Autodesk Fusion 360 part; units mm, degrees
note: some values were not read from the file. Chosen so that the rebuilt part matches the saved one: a direction. Set by a fixed rule: which sketch regions a step uses.
(part 2 of 6)
  spline S11 degree 5 poles (24.2977, -44.2586) (24.3025, -44.2616) (24.312, -44.2677) (24.3261, -44.2771) (24.3444, -44.2904) (24.3667, -44.3078) (24.3886, -44.326) (24.4101, -44.3445) (24.4315, -44.3633) (24.4529, -44.3822) (24.4741, -44.4013) (24.4952, -44.4206) (24.5161, -44.4401) (24.5367, -44.46) (24.5572, -44.4802) (24.5774, -44.5007) (24.5975, -44.5214) (24.6174, -44.5424) (24.6372, -44.5635) (24.6568, -44.5848) (24.6763, -44.6063) (24.6957, -44.6279) (24.715, -44.6497) (24.7341, -44.6718) (24.753, -44.694) (24.7719, -44.7164) (24.7905, -44.739) (24.8091, -44.7617) (24.8275, -44.7846) (24.8458, -44.8077) (24.864, -44.8309) (24.8821, -44.8542) (24.9, -44.8777) (24.9178, -44.9014) (24.9355, -44.9252) (24.9531, -44.9492) (24.9706, -44.9733) (24.9879, -44.9975) (25.0051, -45.0219) (25.0223, -45.0464) (25.0393, -45.0711) (25.0561, -45.0959) (25.0729, -45.1208) (25.0896, -45.1459) (25.1061, -45.171) (25.1225, -45.1963) (25.1389, -45.2218) (25.1551, -45.2473) (25.1712, -45.273) (25.1872, -45.2988) (25.203, -45.3247) (25.2188, -45.3508) (25.2345, -45.3769) (25.25, -45.4032) (25.2655, -45.4296) (25.2808, -45.4561) (25.2961, -45.4827) (25.3112, -45.5094) (25.3262, -45.5363) (25.3411, -45.5632) (25.3559, -45.5903) (25.3706, -45.6175) (25.3852, -45.6447) (25.3997, -45.6721) (25.4141, -45.6996) (25.4284, -45.7272) (25.4426, -45.7549) (25.4566, -45.7827) (25.4706, -45.8106) (25.4845, -45.8386) (25.4982, -45.8667) (25.5092, -45.8892) (25.5173, -45.9062) (25.5227, -45.9175) (25.5254, -45.9232) knots 0 0 0 0 0 0 0.01428571 0.02857143 0.04285714 0.05714286 0.07142857 0.08571429 0.1 0.11428571 0.12857143 0.14285714 0.15714286 0.17142857 0.18571429 0.2 0.21428571 0.22857143 0.24285714 0.25714286 0.27142857 0.28571429 0.3 0.31428571 0.32857143 0.34285714 0.35714286 0.37142857 0.38571429 0.4 0.41428571 0.42857143 0.44285714 0.45714286 0.47142857 0.48571429 0.5 0.51428571 0.52857143 0.54285714 0.55714286 0.57142857 0.58571429 0.6 0.61428571 0.62857143 0.64285714 0.65714286 0.67142857 0.68571429 0.7 0.71428571 0.72857143 0.74285714 0.75714286 0.77142857 0.78571429 0.8 0.81428571 0.82857143 0.84285714 0.85714286 0.87142857 0.88571429 0.9 0.91428571 0.92857143 0.94285714 0.95714286 0.97142857 0.98571429 1 1 1 1 1 1
  line L11 (24.2977, -44.2586) -> (23.8833, -44.0024)
  arc A23 (23.8504, -43.8655) -> (23.8833, -44.0024) centre (23.9359, -43.9173) ccw
  arc A24 (23.8504, -43.8655) -> (24.3428, -42.9686) centre (13.5, -37.5997) ccw
  arc A25 (24.4759, -42.923) -> (24.3428, -42.9686) centre (24.4324, -43.013) ccw
  line L12 (24.4759, -42.923) -> (24.9145, -43.135)
  spline S12 degree 5 poles (24.9145, -43.135) (24.9196, -43.1374) (24.9299, -43.1422) (24.9454, -43.149) (24.9664, -43.1574) (24.9931, -43.1668) (25.0201, -43.1755) (25.0473, -43.1838) (25.0747, -43.1918) (25.1021, -43.1996) (25.1296, -43.2072) (25.1572, -43.2147) (25.1849, -43.2218) (25.2128, -43.2286) (25.2408, -43.235) (25.2689, -43.2411) (25.2972, -43.2469) (25.3255, -43.2524) (25.354, -43.2578) (25.3825, -43.2629) (25.4111, -43.2679) (25.4398, -43.2726) (25.4685, -43.2771) (25.4974, -43.2814) (25.5263, -43.2855) (25.5553, -43.2893) (25.5844, -43.293) (25.6135, -43.2964) (25.6427, -43.2997) (25.672, -43.3027) (25.7014, -43.3056) (25.7308, -43.3083) (25.7602, -43.3108) (25.7898, -43.3132) (25.8194, -43.3153) (25.849, -43.3173) (25.8787, -43.3191) (25.9085, -43.3207) (25.9383, -43.3221) (25.9682, -43.3234) (25.9981, -43.3245) (26.0281, -43.3254) (26.0581, -43.3262) (26.0882, -43.3268) (26.1183, -43.3273) (26.1485, -43.3275) (26.1787, -43.3276) (26.209, -43.3276) (26.2393, -43.3274) (26.2696, -43.327) (26.3, -43.3265) (26.3305, -43.3259) (26.3609, -43.325) (26.3915, -43.3241) (26.422, -43.3229) (26.4526, -43.3216) (26.4832, -43.3202) (26.5139, -43.3186) (26.5446, -43.3169) (26.5754, -43.315) (26.6061, -43.313) (26.637, -43.3108) (26.6678, -43.3085) (26.6987, -43.306) (26.7296, -43.3034) (26.7605, -43.3006) (26.7915, -43.2977) (26.8225, -43.2947) (26.8536, -43.2915) (26.8846, -43.2881) (26.9157, -43.2847) (26.9406, -43.2818) (26.9593, -43.2795) (26.9718, -43.278) (26.978, -43.2772) knots 0 0 0 0 0 0 0.01428571 0.02857143 0.04285714 0.05714286 0.07142857 0.08571429 0.1 0.11428571 0.12857143 0.14285714 0.15714286 0.17142857 0.18571429 0.2 0.21428571 0.22857143 0.24285714 0.25714286 0.27142857 0.28571429 0.3 0.31428571 0.32857143 0.34285714 0.35714286 0.37142857 0.38571429 0.4 0.41428571 0.42857143 0.44285714 0.45714286 0.47142857 0.48571429 0.5 0.51428571 0.52857143 0.54285714 0.55714286 0.57142857 0.58571429 0.6 0.61428571 0.62857143 0.64285714 0.65714286 0.67142857 0.68571429 0.7 0.71428571 0.72857143 0.74285714 0.75714286 0.77142857 0.78571429 0.8 0.81428571 0.82857143 0.84285714 0.85714286 0.87142857 0.88571429 0.9 0.91428571 0.92857143 0.94285714 0.95714286 0.97142857 0.98571429 1 1 1 1 1 1
  arc A26 (26.978, -43.2772) -> (27.2699, -42.5272) centre (13.5, -37.5997) ccw
  spline S13 degree 5 poles (25.6532, -41.2371) (25.6586, -41.2387) (25.6694, -41.2421) (25.6854, -41.2476) (25.7066, -41.2557) (25.7326, -41.2668) (25.7584, -41.2786) (25.784, -41.2909) (25.8096, -41.3035) (25.8351, -41.3163) (25.8605, -41.3292) (25.8859, -41.3424) (25.9111, -41.3559) (25.9362, -41.3697) (25.9612, -41.3839) (25.9861, -41.3985) (26.0108, -41.4133) (26.0355, -41.4284) (26.06, -41.4437) (26.0845, -41.4592) (26.1089, -41.4749) (26.1333, -41.4908) (26.1575, -41.5069) (26.1817, -41.5232) (26.2057, -41.5398) (26.2297, -41.5565) (26.2536, -41.5735) (26.2774, -41.5907) (26.3011, -41.608) (26.3248, -41.6255) (26.3484, -41.6433) (26.3719, -41.6611) (26.3953, -41.6792) (26.4186, -41.6975) (26.4419, -41.7159) (26.465, -41.7345) (26.4881, -41.7532) (26.5112, -41.7722) (26.5341, -41.7913) (26.557, -41.8105) (26.5798, -41.8299) (26.6025, -41.8495) (26.6252, -41.8692) (26.6477, -41.8891) (26.6702, -41.9092) (26.6927, -41.9294) (26.715, -41.9497) (26.7373, -41.9702) (26.7595, -41.9908) (26.7816, -42.0116) (26.8036, -42.0325) (26.8256, -42.0536) (26.8475, -42.0748) (26.8693, -42.0962) (26.8911, -42.1177) (26.9128, -42.1393) (26.9344, -42.1611) (26.9559, -42.183) (26.9774, -42.205) (26.9987, -42.2272) (27.0201, -42.2495) (27.0413, -42.2719) (27.0624, -42.2945) (27.0835, -42.3172) (27.1045, -42.34) (27.1255, -42.363) (27.1463, -42.386) (27.1671, -42.4092) (27.1878, -42.4326) (27.2085, -42.456) (27.229, -42.4796) (27.2454, -42.4986) (27.2577, -42.5128) (27.2659, -42.5224) (27.2699, -42.5272) knots 0 0 0 0 0 0 0.01428571 0.02857143 0.04285714 0.05714286 0.07142857 0.08571429 0.1 0.11428571 0.12857143 0.14285714 0.15714286 0.17142857 0.18571429 0.2 0.21428571 0.22857143 0.24285714 0.25714286 0.27142857 0.28571429 0.3 0.31428571 0.32857143 0.34285714 0.35714286 0.37142857 0.38571429 0.4 0.41428571 0.42857143 0.44285714 0.45714286 0.47142857 0.48571429 0.5 0.51428571 0.52857143 0.54285714 0.55714286 0.57142857 0.58571429 0.6 0.61428571 0.62857143 0.64285714 0.65714286 0.67142857 0.68571429 0.7 0.71428571 0.72857143 0.74285714 0.75714286 0.77142857 0.78571429 0.8 0.81428571 0.82857143 0.84285714 0.85714286 0.87142857 0.88571429 0.9 0.91428571 0.92857143 0.94285714 0.95714286 0.97142857 0.98571429 1 1 1 1 1 1
  line L13 (25.6532, -41.2371) -> (25.1866, -41.0968)
  arc A27 (25.1194, -40.9731) -> (25.1866, -41.0968) centre (25.2154, -41.001) ccw
  arc A28 (25.1194, -40.9731) -> (25.3629, -39.9794) centre (13.5, -37.5997) ccw
  arc A29 (25.4796, -39.9008) -> (25.3629, -39.9794) centre (25.4609, -39.999) ccw
  line L14 (25.4796, -39.9008) -> (25.9582, -39.9921)
  spline S14 degree 5 poles (25.9582, -39.9921) (25.9638, -39.9931) (25.9749, -39.9951) (25.9917, -39.9977) (26.0141, -40.0003) (26.0424, -40.0025) (26.0707, -40.0039) (26.0991, -40.0048) (26.1276, -40.0055) (26.1561, -40.0059) (26.1847, -40.0062) (26.2132, -40.0062) (26.2419, -40.006) (26.2705, -40.0053) (26.2992, -40.0042) (26.328, -40.0028) (26.3568, -40.0011) (26.3856, -39.9991) (26.4145, -39.9969) (26.4434, -39.9945) (26.4723, -39.9919) (26.5012, -39.989) (26.5301, -39.986) (26.5591, -39.9827) (26.5881, -39.9791) (26.6171, -39.9753) (26.6461, -39.9713) (26.6752, -39.9671) (26.7042, -39.9627) (26.7333, -39.958) (26.7624, -39.9532) (26.7915, -39.9482) (26.8206, -39.943) (26.8498, -39.9376) (26.8789, -39.9321) (26.908, -39.9263) (26.9372, -39.9203) (26.9664, -39.9142) (26.9956, -39.9079) (27.0247, -39.9014) (27.0539, -39.8947) (27.0831, -39.8878) (27.1123, -39.8808) (27.1415, -39.8736) (27.1708, -39.8662) (27.2, -39.8587) (27.2292, -39.851) (27.2584, -39.8431) (27.2876, -39.8351) (27.3169, -39.8269) (27.3461, -39.8185) (27.3753, -39.81) (27.4045, -39.8013) (27.4338, -39.7924) (27.463, -39.7834) (27.4922, -39.7743) (27.5214, -39.765) (27.5506, -39.7555) (27.5798, -39.7459) (27.6091, -39.7361) (27.6383, -39.7262) (27.6675, -39.7161) (27.6967, -39.7059) (27.7258, -39.6955) (27.755, -39.6849) (27.7842, -39.6743) (27.8134, -39.6634) (27.8425, -39.6525) (27.8717, -39.6414) (27.9008, -39.6301) (27.93, -39.6187) (27.9533, -39.6095) (27.9707, -39.6025) (27.9824, -39.5978) (27.9882, -39.5954) knots 0 0 0 0 0 0 0.01428571 0.02857143 0.04285714 0.05714286 0.07142857 0.08571429 0.1 0.11428571 0.12857143 0.14285714 0.15714286 0.17142857 0.18571429 0.2 0.21428571 0.22857143 0.24285714 0.25714286 0.27142857 0.28571429 0.3 0.31428571 0.32857143 0.34285714 0.35714286 0.37142857 0.38571429 0.4 0.41428571 0.42857143 0.44285714 0.45714286 0.47142857 0.48571429 0.5 0.51428571 0.52857143 0.54285714 0.55714286 0.57142857 0.58571429 0.6 0.61428571 0.62857143 0.64285714 0.65714286 0.67142857 0.68571429 0.7 0.71428571 0.72857143 0.74285714 0.75714286 0.77142857 0.78571429 0.8 0.81428571 0.82857143 0.84285714 0.85714286 0.87142857 0.88571429 0.9 0.91428571 0.92857143 0.94285714 0.95714286 0.97142857 0.98571429 1 1 1 1 1 1
  arc A30 (27.9882, -39.5954) -> (28.076, -38.7953) centre (13.5, -37.5997) ccw
  spline S15 degree 5 poles (26.1805, -37.9677) (26.1862, -37.9679) (26.1975, -37.9683) (26.2144, -37.9695) (26.2369, -37.9718) (26.2649, -37.9758) (26.2929, -37.9805) (26.3208, -37.9858) (26.3488, -37.9913) (26.3767, -37.9971) (26.4046, -38.003) (26.4325, -38.0092) (26.4604, -38.0157) (26.4882, -38.0225) (26.516, -38.0298) (26.5438, -38.0374) (26.5716, -38.0453) (26.5993, -38.0535) (26.627, -38.0619) (26.6546, -38.0706) (26.6823, -38.0794) (26.7099, -38.0884) (26.7375, -38.0977) (26.765, -38.1073) (26.7925, -38.117) (26.82, -38.127) (26.8475, -38.1372) (26.875, -38.1476) (26.9024, -38.1583) (26.9297, -38.1691) (26.9571, -38.1801) (26.9844, -38.1913) (27.0117, -38.2027) (27.039, -38.2143) (27.0662, -38.226) (27.0934, -38.238) (27.1206, -38.2501) (27.1477, -38.2625) (27.1749, -38.275) (27.2019, -38.2876) (27.229, -38.3005) (27.256, -38.3135) (27.283, -38.3267) (27.3099, -38.3401) (27.3368, -38.3536) (27.3637, -38.3673) (27.3906, -38.3812) (27.4174, -38.3952) (27.4442, -38.4094) (27.4709, -38.4237) (27.4976, -38.4383) (27.5243, -38.4529) (27.551, -38.4677) (27.5776, -38.4827) (27.6041, -38.4978) (27.6307, -38.5131) (27.6572, -38.5286) (27.6836, -38.5441) (27.7101, -38.5599) (27.7365, -38.5758) (27.7628, -38.5918) (27.7891, -38.608) (27.8154, -38.6243) (27.8417, -38.6408) (27.8679, -38.6574) (27.894, -38.6741) (27.9201, -38.691) (27.9462, -38.708) (27.9723, -38.7252) (27.9983, -38.7425) (28.0242, -38.76) (28.045, -38.7741) (28.0605, -38.7847) (28.0709, -38.7918) (28.076, -38.7953) knots 0 0 0 0 0 0 0.01428571 0.02857143 0.04285714 0.05714286 0.07142857 0.08571429 0.1 0.11428571 0.12857143 0.14285714 0.15714286 0.17142857 0.18571429 0.2 0.21428571 0.22857143 0.24285714 0.25714286 0.27142857 0.28571429 0.3 0.31428571 0.32857143 0.34285714 0.35714286 0.37142857 0.38571429 0.4 0.41428571 0.42857143 0.44285714 0.45714286 0.47142857 0.48571429 0.5 0.51428571 0.52857143 0.54285714 0.55714286 0.57142857 0.58571429 0.6 0.61428571 0.62857143 0.64285714 0.65714286 0.67142857 0.68571429 0.7 0.71428571 0.72857143 0.74285714 0.75714286 0.77142857 0.78571429 0.8 0.81428571 0.82857143 0.84285714 0.85714286 0.87142857 0.88571429 0.9 0.91428571 0.92857143 0.94285714 0.95714286 0.97142857 0.98571429 1 1 1 1 1 1
  line L15 (26.1805, -37.9677) -> (25.6935, -37.9529)
  arc A31 (25.5966, -37.8509) -> (25.6935, -37.9529) centre (25.6966, -37.853) ccw
  arc A32 (25.5966, -37.8509) -> (25.5746, -36.828) centre (13.5, -37.5997) ccw
  arc A33 (25.667, -36.7218) -> (25.5746, -36.828) centre (25.6744, -36.8216) ccw
  line L16 (25.667, -36.7218) -> (26.1529, -36.6861)
  spline S16 degree 5 poles (26.1529, -36.6861) (26.1586, -36.6857) (26.1698, -36.6847) (26.1867, -36.6829) (26.209, -36.6796) (26.2369, -36.6744) (26.2646, -36.6684) (26.2923, -36.662) (26.32, -36.6552) (26.3476, -36.6483) (26.3753, -36.6412) (26.4029, -36.6338) (26.4305, -36.6261) (26.458, -36.6181) (26.4855, -36.6096) (26.5129, -36.6008) (26.5402, -36.5917) (26.5676, -36.5823) (26.5949, -36.5727) (26.6221, -36.5629) (26.6494, -36.5529) (26.6766, -36.5427) (26.7037, -36.5322) (26.7309, -36.5215) (26.7579, -36.5106) (26.785, -36.4994) (26.812, -36.488) (26.839, -36.4764) (26.8659, -36.4646) (26.8928, -36.4527) (26.9196, -36.4405) (26.9465, -36.4281) (26.9732, -36.4156) (27, -36.4028) (27.0267, -36.3899) (27.0533, -36.3768) (27.08, -36.3634) (27.1066, -36.35) (27.1331, -36.3363) (27.1596, -36.3225) (27.1861, -36.3085) (27.2125, -36.2943) (27.2389, -36.2799) (27.2652, -36.2654) (27.2916, -36.2508) (27.3178, -36.2359) (27.344, -36.2209) (27.3702, -36.2057) (27.3964, -36.1904) (27.4225, -36.1749) (27.4486, -36.1593) (27.4746, -36.1435) (27.5006, -36.1275) (27.5265, -36.1114) (27.5524, -36.0952) (27.5782, -36.0787) (27.6041, -36.0622) (27.6298, -36.0455) (27.6556, -36.0286) (27.6812, -36.0116) (27.7069, -35.9945) (27.7325, -35.9772) (27.758, -35.9597) (27.7835, -35.9421) (27.809, -35.9244) (27.8344, -35.9066) (27.8598, -35.8886) (27.8851, -35.8704) (27.9104, -35.8521) (27.9356, -35.8337) (27.9608, -35.8152) (27.9809, -35.8002) (27.996, -35.7889) (28.006, -35.7814) (28.011, -35.7776) knots 0 0 0 0 0 0 0.01428571 0.02857143 0.04285714 0.05714286 0.07142857 0.08571429 0.1 0.11428571 0.12857143 0.14285714 0.15714286 0.17142857 0.18571429 0.2 0.21428571 0.22857143 0.24285714 0.25714286 0.27142857 0.28571429 0.3 0.31428571 0.32857143 0.34285714 0.35714286 0.37142857 0.38571429 0.4 0.41428571 0.42857143 0.44285714 0.45714286 0.47142857 0.48571429 0.5 0.51428571 0.52857143 0.54285714 0.55714286 0.57142857 0.58571429 0.6 0.61428571 0.62857143 0.64285714 0.65714286 0.67142857 0.68571429 0.7 0.71428571 0.72857143 0.74285714 0.75714286 0.77142857 0.78571429 0.8 0.81428571 0.82857143 0.84285714 0.85714286 0.87142857 0.88571429 0.9 0.91428571 0.92857143 0.94285714 0.95714286 0.97142857 0.98571429 1 1 1 1 1 1
  arc A34 (28.011, -35.7776) -> (27.8888, -34.982) centre (13.5, -37.5997) ccw
  spline S17 degree 5 poles (25.8437, -34.6732) (25.8492, -34.6719) (25.8602, -34.6694) (25.8769, -34.6662) (25.8992, -34.6626) (25.9273, -34.6591) (25.9555, -34.6565) (25.9839, -34.6544) (26.0123, -34.6525) (26.0408, -34.6508) (26.0693, -34.6493) (26.0978, -34.648) (26.1264, -34.6471) (26.1551, -34.6465) (26.1838, -34.6463) (26.2126, -34.6465) (26.2415, -34.647) (26.2704, -34.6477) (26.2993, -34.6487) (26.3282, -34.6498) (26.3572, -34.6512) (26.3862, -34.6528) (26.4153, -34.6546) (26.4444, -34.6567) (26.4735, -34.659) (26.5026, -34.6616) (26.5318, -34.6643) (26.561, -34.6673) (26.5903, -34.6704) (26.6195, -34.6738) (26.6488, -34.6773) (26.6781, -34.6811) (26.7074, -34.685) (26.7367, -34.6892) (26.7661, -34.6935) (26.7954, -34.698) (26.8248, -34.7027) (26.8542, -34.7076) (26.8837, -34.7126) (26.9131, -34.7179) (26.9426, -34.7233) (26.972, -34.7289) (27.0015, -34.7347) (27.031, -34.7406) (27.0605, -34.7467) (27.09, -34.753) (27.1195, -34.7594) (27.1491, -34.766) (27.1786, -34.7728) (27.2082, -34.7797) (27.2377, -34.7868) (27.2673, -34.7941) (27.2968, -34.8015) (27.3264, -34.8091) (27.356, -34.8168) (27.3856, -34.8247) (27.4152, -34.8328) (27.4448, -34.841) (27.4744, -34.8493) (27.504, -34.8578) (27.5336, -34.8665) (27.5632, -34.8753) (27.5928, -34.8843) (27.6224, -34.8934) (27.652, -34.9027) (27.6816, -34.9121) (27.7112, -34.9216) (27.7408, -34.9313) (27.7704, -34.9412) (27.8, -34.9512) (27.8296, -34.9613) (27.8533, -34.9695) (27.8711, -34.9758) (27.8829, -34.9799) (27.8888, -34.982) knots 0 0 0 0 0 0 0.01428571 0.02857143 0.04285714 0.05714286 0.07142857 0.08571429 0.1 0.11428571 0.12857143 0.14285714 0.15714286 0.17142857 0.18571429 0.2 0.21428571 0.22857143 0.24285714 0.25714286 0.27142857 0.28571429 0.3 0.31428571 0.32857143 0.34285714 0.35714286 0.37142857 0.38571429 0.4 0.41428571 0.42857143 0.44285714 0.45714286 0.47142857 0.48571429 0.5 0.51428571 0.52857143 0.54285714 0.55714286 0.57142857 0.58571429 0.6 0.61428571 0.62857143 0.64285714 0.65714286 0.67142857 0.68571429 0.7 0.71428571 0.72857143 0.74285714 0.75714286 0.77142857 0.78571429 0.8 0.81428571 0.82857143 0.84285714 0.85714286 0.87142857 0.88571429 0.9 0.91428571 0.92857143 0.94285714 0.95714286 0.97142857 0.98571429 1 1 1 1 1 1
  line L17 (25.8437, -34.6732) -> (25.3695, -34.785)
  arc A35 (25.2494, -34.7115) -> (25.3695, -34.785) centre (25.3465, -34.6876) ccw
  arc A36 (25.2494, -34.7115) -> (24.9634, -33.7291) centre (13.5, -37.5997) ccw
  arc A37 (25.0252, -33.6027) -> (24.9634, -33.7291) centre (25.0581, -33.6971) ccw
  line L18 (25.0252, -33.6027) -> (25.4853, -33.4424)
  spline S18 degree 5 poles (25.4853, -33.4424) (25.4907, -33.4406) (25.5013, -33.4367) (25.5171, -33.4305) (25.5378, -33.4216) (25.5634, -33.4094) (25.5887, -33.3964) (25.6137, -33.383) (25.6387, -33.3694) (25.6636, -33.3555) (25.6885, -33.3415) (25.7133, -33.3272) (25.7379, -33.3127) (25.7624, -33.2977) (25.7867, -33.2825) (25.8109, -33.2669) (25.835, -33.251) (25.859, -33.2349) (25.8829, -33.2185) (25.9067, -33.202) (25.9304, -33.1853) (25.954, -33.1683) (25.9775, -33.1512) (26.001, -33.1339) (26.0243, -33.1163) (26.0475, -33.0985) (26.0707, -33.0805) (26.0937, -33.0623) (26.1167, -33.044) (26.1396, -33.0254) (26.1623, -33.0067) (26.185, -32.9878) (26.2077, -32.9688) (26.2302, -32.9495) (26.2526, -32.9301) (26.275, -32.9106) (26.2973, -32.8908) (26.3195, -32.8709) (26.3416, -32.8508) (26.3636, -32.8306) (26.3855, -32.8102) (26.4074, -32.7897) (26.4292, -32.769) (26.4509, -32.7482) (26.4725, -32.7272) (26.494, -32.7061) (26.5155, -32.6848) (26.5368, -32.6633) (26.5581, -32.6418) (26.5793, -32.6201) (26.6005, -32.5982) (26.6215, -32.5762) (26.6425, -32.5541) (26.6634, -32.5318) (26.6842, -32.5094) (26.7049, -32.4868) (26.7255, -32.4642) (26.7461, -32.4414) (26.7666, -32.4184) (26.787, -32.3953) (26.8073, -32.3721) (26.8276, -32.3488) (26.8477, -32.3254) (26.8678, -32.3018) (26.8878, -32.2781) (26.9078, -32.2542) (26.9276, -32.2303) (26.9474, -32.2062) (26.9671, -32.182) (26.9867, -32.1577) (27.0062, -32.1332) (27.0218, -32.1136) (27.0334, -32.0988) (27.0411, -32.0889) (27.045, -32.084) knots 0 0 0 0 0 0 0.01428571 0.02857143 0.04285714 0.05714286 0.07142857 0.08571429 0.1 0.11428571 0.12857143 0.14285714 0.15714286 0.17142857 0.18571429 0.2 0.21428571 0.22857143 0.24285714 0.25714286 0.27142857 0.28571429 0.3 0.31428571 0.32857143 0.34285714 0.35714286 0.37142857 0.38571429 0.4 0.41428571 0.42857143 0.44285714 0.45714286 0.47142857 0.48571429 0.5 0.51428571 0.52857143 0.54285714 0.55714286 0.57142857 0.58571429 0.6 0.61428571 0.62857143 0.64285714 0.65714286 0.67142857 0.68571429 0.7 0.71428571 0.72857143 0.74285714 0.75714286 0.77142857 0.78571429 0.8 0.81428571 0.82857143 0.84285714 0.85714286 0.87142857 0.88571429 0.9 0.91428571 0.92857143 0.94285714 0.95714286 0.97142857 0.98571429 1 1 1 1 1 1
  arc A38 (27.045, -32.084) -> (26.721, -31.3471) centre (13.5, -37.5997) ccw
  spline S19 degree 5 poles (24.6656, -31.5781) (24.6706, -31.5755) (24.6806, -31.5702) (24.6959, -31.5628) (24.7165, -31.5535) (24.7428, -31.5429) (24.7694, -31.5331) (24.7962, -31.5237) (24.8232, -31.5145) (24.8502, -31.5055) (24.8774, -31.4967) (24.9046, -31.4881) (24.932, -31.4797) (24.9596, -31.4718) (24.9873, -31.4642) (25.0151, -31.4569) (25.0431, -31.4499) (25.0712, -31.4431) (25.0994, -31.4365) (25.1277, -31.4302) (25.156, -31.424) (25.1844, -31.418) (25.213, -31.4123) (25.2416, -31.4067) (25.2703, -31.4014) (25.2991, -31.3963) (25.328, -31.3914) (25.357, -31.3868) (25.3861, -31.3822) (25.4152, -31.3779) (25.4444, -31.3738) (25.4736, -31.3698) (25.503, -31.366) (25.5324, -31.3624) (25.5619, -31.359) (25.5914, -31.3558) (25.621, -31.3527) (25.6507, -31.3498) (25.6804, -31.3471) (25.7102, -31.3445) (25.74, -31.3421) (25.7699, -31.3399) (25.7999, -31.3378) (25.8299, -31.3359) (25.86, -31.3342) (25.8901, -31.3326) (25.9203, -31.3312) (25.9506, -31.3299) (25.9809, -31.3288) (26.0112, -31.3279) (26.0416, -31.3271) (26.072, -31.3265) (26.1025, -31.326) (26.133, -31.3256) (26.1636, -31.3254) (26.1942, -31.3254) (26.2249, -31.3255) (26.2556, -31.3258) (26.2864, -31.3262) (26.3172, -31.3268) (26.348, -31.3275) (26.3789, -31.3283) (26.4098, -31.3293) (26.4408, -31.3305) (26.4717, -31.3317) (26.5028, -31.3332) (26.5339, -31.3347) (26.565, -31.3364) (26.5961, -31.3383) (26.6273, -31.3403) (26.6585, -31.3424) (26.6835, -31.3442) (26.7023, -31.3457) (26.7148, -31.3466) (26.721, -31.3471) knots 0 0 0 0 0 0 0.01428571 0.02857143 0.04285714 0.05714286 0.07142857 0.08571429 0.1 0.11428571 0.12857143 0.14285714 0.15714286 0.17142857 0.18571429 0.2 0.21428571 0.22857143 0.24285714 0.25714286 0.27142857 0.28571429 0.3 0.31428571 0.32857143 0.34285714 0.35714286 0.37142857 0.38571429 0.4 0.41428571 0.42857143 0.44285714 0.45714286 0.47142857 0.48571429 0.5 0.51428571 0.52857143 0.54285714 0.55714286 0.57142857 0.58571429 0.6 0.61428571 0.62857143 0.64285714 0.65714286 0.67142857 0.68571429 0.7 0.71428571 0.72857143 0.74285714 0.75714286 0.77142857 0.78571429 0.8 0.81428571 0.82857143 0.84285714 0.85714286 0.87142857 0.88571429 0.9 0.91428571 0.92857143 0.94285714 0.95714286 0.97142857 0.98571429 1 1 1 1 1 1
  line L19 (24.6656, -31.5781) -> (24.2365, -31.8088)
  arc A39 (24.1015, -31.7689) -> (24.2365, -31.8088) centre (24.1892, -31.7207) ccw
  arc A40 (24.1015, -31.7689) -> (23.571, -30.8941) centre (13.5, -37.5997) ccw
  arc A41 (23.598, -30.7559) -> (23.571, -30.8941) centre (23.6542, -30.8387) ccw
  line L20 (23.598, -30.7559) -> (24.0009, -30.4821)
  spline S20 degree 5 poles (24.0009, -30.4821) (24.0056, -30.4789) (24.0149, -30.4724) (24.0286, -30.4624) (24.0463, -30.4483) (24.0678, -30.4299) (24.0889, -30.4109) (24.1096, -30.3915) (24.1302, -30.3718) (24.1507, -30.3519) (24.1711, -30.332) (24.1913, -30.3118) (24.2113, -30.2913) (24.2311, -30.2706) (24.2507, -30.2495) (24.27, -30.2282) (24.2892, -30.2066) (24.3082, -30.1848) (24.327, -30.1629) (24.3457, -30.1408) (24.3643, -30.1185) (24.3827, -30.096) (24.401, -30.0734) (24.4192, -30.0505) (24.4371, -30.0275) (24.455, -30.0043) (24.4727, -29.981) (24.4902, -29.9574) (24.5077, -29.9338) (24.525, -29.9099) (24.5421, -29.886) (24.5592, -29.8619) (24.5761, -29.8376) (24.5929, -29.8132) (24.6095, -29.7886) (24.6261, -29.7639) (24.6425, -29.7391) (24.6587, -29.7141) (24.6749, -29.689) (24.6909, -29.6638) (24.7069, -29.6384) (24.7227, -29.6129) (24.7383, -29.5873) (24.7539, -29.5616) (24.7694, -29.5357) (24.7847, -29.5097) (24.7999, -29.4836) (24.815, -29.4574) (24.83, -29.431) (24.8448, -29.4046) (24.8596, -29.378) (24.8742, -29.3513) (24.8887, -29.3245) (24.9031, -29.2976) (24.9174, -29.2705) (24.9316, -29.2434) (24.9457, -29.2161) (24.9597, -29.1888) (24.9735, -29.1613) (24.9873, -29.1338) (25.0009, -29.1061) (25.0144, -29.0783) (25.0278, -29.0504) (25.0411, -29.0225) (25.0543, -28.9944) (25.0674, -28.9662) (25.0804, -28.9379) (25.0932, -28.9095) (25.106, -28.8811) (25.1186, -28.8525) (25.1312, -28.8238) (25.1411, -28.8008) (25.1485, -28.7835) (25.1534, -28.772) (25.1559, -28.7662) knots 0 0 0 0 0 0 0.01428571 0.02857143 0.04285714 0.05714286 0.07142857 0.08571429 0.1 0.11428571 0.12857143 0.14285714 0.15714286 0.17142857 0.18571429 0.2 0.21428571 0.22857143 0.24285714 0.25714286 0.27142857 0.28571429 0.3 0.31428571 0.32857143 0.34285714 0.35714286 0.37142857 0.38571429 0.4 0.41428571 0.42857143 0.44285714 0.45714286 0.47142857 0.48571429 0.5 0.51428571 0.52857143 0.54285714 0.55714286 0.57142857 0.58571429 0.6 0.61428571 0.62857143 0.64285714 0.65714286 0.67142857 0.68571429 0.7 0.71428571 0.72857143 0.74285714 0.75714286 0.77142857 0.78571429 0.8 0.81428571 0.82857143 0.84285714 0.85714286 0.87142857 0.88571429 0.9 0.91428571 0.92857143 0.94285714 0.95714286 0.97142857 0.98571429 1 1 1 1 1 1
  arc A42 (25.1559, -28.7662) -> (24.6523, -28.1383) centre (13.5, -37.5997) ccw
  spline S21 degree 5 poles (22.7267, -28.8934) (22.7308, -28.8896) (22.7391, -28.8819) (22.7519, -28.8708) (22.7694, -28.8565) (22.7921, -28.8395) (22.8152, -28.8231) (22.8387, -28.807) (22.8624, -28.7912) (22.8862, -28.7755) (22.9101, -28.7599) (22.9342, -28.7446) (22.9585, -28.7295) (22.9831, -28.7146) (23.0078, -28.7001) (23.0329, -28.6858) (23.0581, -28.6718) (23.0835, -28.658) (23.109, -28.6444) (23.1347, -28.6309) (23.1604, -28.6176) (23.1864, -28.6045) (23.2124, -28.5916) (23.2387, -28.5788) (23.265, -28.5663) (23.2915, -28.5539) (23.3182, -28.5417) (23.345, -28.5296) (23.3719, -28.5178) (23.3989, -28.506) (23.426, -28.4945) (23.4532, -28.4831) (23.4806, -28.4718) (23.5081, -28.4607) (23.5356, -28.4498) (23.5633, -28.439) (23.5911, -28.4284) (23.619, -28.4179) (23.6471, -28.4076) (23.6752, -28.3974) (23.7034, -28.3874) (23.7317, -28.3775) (23.7601, -28.3678) (23.7886, -28.3581) (23.8172, -28.3487) (23.8459, -28.3394) (23.8747, -28.3302) (23.9036, -28.3211) (23.9326, -28.3122) (23.9616, -28.3035) (23.9908, -28.2948) (24.02, -28.2863) (24.0493, -28.278) (24.0787, -28.2697) (24.1082, -28.2617) (24.1378, -28.2537) (24.1674, -28.2459) (24.1972, -28.2382) (24.227, -28.2306) (24.2569, -28.2232) (24.2868, -28.2159) (24.3169, -28.2087) (24.347, -28.2017) (24.3772, -28.1948) (24.4075, -28.188) (24.4378, -28.1813) (24.4682, -28.1748) (24.4987, -28.1684) (24.5293, -28.1621) (24.5599, -28.156) (24.5906, -28.15) (24.6152, -28.1452) (24.6337, -28.1418) (24.6461, -28.1395) (24.6523, -28.1383) knots 0 0 0 0 0 0 0.01428571 0.02857143 0.04285714 0.05714286 0.07142857 0.08571429 0.1 0.11428571 0.12857143 0.14285714 0.15714286 0.17142857 0.18571429 0.2 0.21428571 0.22857143 0.24285714 0.25714286 0.27142857 0.28571429 0.3 0.31428571 0.32857143 0.34285714 0.35714286 0.37142857 0.38571429 0.4 0.41428571 0.42857143 0.44285714 0.45714286 0.47142857 0.48571429 0.5 0.51428571 0.52857143 0.54285714 0.55714286 0.57142857 0.58571429 0.6 0.61428571 0.62857143 0.64285714 0.65714286 0.67142857 0.68571429 0.7 0.71428571 0.72857143 0.74285714 0.75714286 0.77142857 0.78571429 0.8 0.81428571 0.82857143 0.84285714 0.85714286 0.87142857 0.88571429 0.9 0.91428571 0.92857143 0.94285714 0.95714286 0.97142857 0.98571429 1 1 1 1 1 1
  line L21 (22.7267, -28.8934) -> (22.3719, -29.2273)
  arc A43 (22.2312, -29.2237) -> (22.3719, -29.2273) centre (22.3033, -29.1545) ccw
  arc A44 (22.2312, -29.2237) -> (21.4923, -28.516) centre (13.5, -37.5997) ccw
  arc A45 (21.4826, -28.3756) -> (21.4923, -28.516) centre (21.5583, -28.4409) ccw
  line L22 (21.4826, -28.3756) -> (21.8009, -28.0067)
  spline S22 degree 5 poles (21.8009, -28.0067) (21.8046, -28.0025) (21.8119, -27.9938) (21.8225, -27.9806) (21.836, -27.9624) (21.852, -27.9391) (21.8674, -27.9153) (21.8825, -27.8911) (21.8973, -27.8668) (21.9119, -27.8423) (21.9264, -27.8177) (21.9407, -27.793) (21.9548, -27.7681) (21.9685, -27.7429) (21.982, -27.7175) (21.9952, -27.6919) (22.0081, -27.6661) (22.0208, -27.6401) (22.0333, -27.6141) (22.0456, -27.5878) (22.0578, -27.5615) (22.0698, -27.535) (22.0816, -27.5084) (22.0932, -27.4817) (22.1046, -27.4548) (22.1159, -27.4278) (22.1269, -27.4006) (22.1378, -27.3734) (22.1485, -27.346) (22.159, -27.3185) (22.1694, -27.2909) (22.1796, -27.2632) (22.1897, -27.2354) (22.1996, -27.2075) (22.2093, -27.1794) (22.2189, -27.1513) (22.2283, -27.1231) (22.2376, -27.0947) (22.2467, -27.0663) (22.2557, -27.0378) (22.2645, -27.0091) (22.2731, -26.9804) (22.2816, -26.9516) (22.29, -26.9227) (22.2982, -26.8938) (22.3063, -26.8647) (22.3142, -26.8355) (22.322, -26.8063) (22.3297, -26.777) (22.3372, -26.7475) (22.3446, -26.7181) (22.3518, -26.6885) (22.3589, -26.6588) (22.3658, -26.6291) (22.3727, -26.5993) (22.3793, -26.5694) (22.3859, -26.5394) (22.3923, -26.5094) (22.3985, -26.4793) (22.4047, -26.4491) (22.4107, -26.4189) (22.4166, -26.3885) (22.4223, -26.3581) (22.4279, -26.3277) (22.4334, -26.2971) (22.4387, -26.2665) (22.4439, -26.2358) (22.449, -26.2051) (22.454, -26.1743) (22.4588, -26.1434) (22.4635, -26.1125) (22.4671, -26.0877) (22.4698, -26.0691) (22.4716, -26.0566) (22.4724, -26.0504) knots 0 0 0 0 0 0 0.01428571 0.02857143 0.04285714 0.05714286 0.07142857 0.08571429 0.1 0.11428571 0.12857143 0.14285714 0.15714286 0.17142857 0.18571429 0.2 0.21428571 0.22857143 0.24285714 0.25714286 0.27142857 0.28571429 0.3 0.31428571 0.32857143 0.34285714 0.35714286 0.37142857 0.38571429 0.4 0.41428571 0.42857143 0.44285714 0.45714286 0.47142857 0.48571429 0.5 0.51428571 0.52857143 0.54285714 0.55714286 0.57142857 0.58571429 0.6 0.61428571 0.62857143 0.64285714 0.65714286 0.67142857 0.68571429 0.7 0.71428571 0.72857143 0.74285714 0.75714286 0.77142857 0.78571429 0.8 0.81428571 0.82857143 0.84285714 0.85714286 0.87142857 0.88571429 0.9 0.91428571 0.92857143 0.94285714 0.95714286 0.97142857 0.98571429 1 1 1 1 1 1
  arc A46 (22.4724, -26.0504) -> (21.8235, -25.5743) centre (13.5, -37.5997) ccw
  spline S23 degree 5 poles (20.1589, -26.8021) (20.1619, -26.7972) (20.168, -26.7877) (20.1774, -26.7736) (20.1907, -26.7553) (20.2081, -26.733) (20.2262, -26.7112) (20.2448, -26.6896) (20.2635, -26.6682) (20.2825, -26.6468) (20.3016, -26.6256) (20.3209, -26.6046) (20.3404, -26.5837) (20.3603, -26.563) (20.3805, -26.5425) (20.401, -26.5223) (20.4217, -26.5022) (20.4426, -26.4823) (20.4638, -26.4625) (20.4851, -26.4429) (20.5065, -26.4234) (20.5282, -26.404) (20.55, -26.3847) (20.572, -26.3656) (20.5943, -26.3467) (20.6167, -26.3279) (20.6392, -26.3092) (20.662, -26.2906) (20.6849, -26.2722) (20.7079, -26.2539) (20.7312, -26.2357) (20.7545, -26.2176) (20.778, -26.1997) (20.8017, -26.1819) (20.8255, -26.1642) (20.8495, -26.1466) (20.8736, -26.1291) (20.8978, -26.1118) (20.9222, -26.0946) (20.9467, -26.0775) (20.9714, -26.0605) (20.9962, -26.0436) (21.0211, -26.0268) (21.0461, -26.0102) (21.0713, -25.9936) (21.0966, -25.9772) (21.1221, -25.9609) (21.1476, -25.9446) (21.1733, -25.9285) (21.1991, -25.9126) (21.225, -25.8967) (21.2511, -25.8809) (21.2772, -25.8652) (21.3035, -25.8497) (21.3299, -25.8342) (21.3564, -25.8189) (21.383, -25.8037) (21.4097, -25.7885) (21.4366, -25.7735) (21.4635, -25.7586) (21.4906, -25.7438) (21.5177, -25.7291) (21.545, -25.7145) (21.5724, -25.7) (21.5999, -25.6856) (21.6275, -25.6713) (21.6552, -25.6572) (21.683, -25.6431) (21.7109, -25.6291) (21.7388, -25.6153) (21.7669, -25.6015) (21.7895, -25.5906) (21.8065, -25.5824) (21.8178, -25.577) (21.8235, -25.5743) knots 0 0 0 0 0 0 0.01428571 0.02857143 0.04285714 0.05714286 0.07142857 0.08571429 0.1 0.11428571 0.12857143 0.14285714 0.15714286 0.17142857 0.18571429 0.2 0.21428571 0.22857143 0.24285714 0.25714286 0.27142857 0.28571429 0.3 0.31428571 0.32857143 0.34285714 0.35714286 0.37142857 0.38571429 0.4 0.41428571 0.42857143 0.44285714 0.45714286 0.47142857 0.48571429 0.5 0.51428571 0.52857143 0.54285714 0.55714286 0.57142857 0.58571429 0.6 0.61428571 0.62857143 0.64285714 0.65714286 0.67142857 0.68571429 0.7 0.71428571 0.72857143 0.74285714 0.75714286 0.77142857 0.78571429 0.8 0.81428571 0.82857143 0.84285714 0.85714286 0.87142857 0.88571429 0.9 0.91428571 0.92857143 0.94285714 0.95714286 0.97142857 0.98571429 1 1 1 1 1 1
  line L23 (20.1589, -26.8021) -> (19.9026, -27.2164)
  arc A47 (19.7658, -27.2493) -> (19.9026, -27.2164) centre (19.8176, -27.1638) ccw
  arc A48 (19.7658, -27.2493) -> (18.8689, -26.757) centre (13.5, -37.5997) ccw
  arc A49 (18.8233, -26.6238) -> (18.8689, -26.757) centre (18.9133, -26.6673) ccw
  line L24 (18.8233, -26.6238) -> (19.0352, -26.1852)
  spline S24 degree 5 poles (19.0352, -26.1852) (19.0377, -26.1801) (19.0425, -26.1698) (19.0493, -26.1543) (19.0577, -26.1333) (19.0671, -26.1066) (19.0758, -26.0796) (19.0841, -26.0524) (19.0921, -26.025) (19.0999, -25.9976) (19.1075, -25.9701) (19.115, -25.9425) (19.1221, -25.9148) (19.1289, -25.8869) (19.1353, -25.8589) (19.1414, -25.8308) (19.1472, -25.8025) (19.1527, -25.7742) (19.158, -25.7457) (19.1632, -25.7172) (19.1681, -25.6886) (19.1729, -25.6599) (19.1774, -25.6312) (19.1817, -25.6023) (19.1857, -25.5734) (19.1896, -25.5444) (19.1932, -25.5153) (19.1967, -25.4862) (19.1999, -25.457) (19.203, -25.4277) (19.2059, -25.3984) (19.2086, -25.3689) (19.2111, -25.3395) (19.2134, -25.3099) (19.2156, -25.2804) (19.2176, -25.2507) (19.2193, -25.221) (19.221, -25.1912) (19.2224, -25.1614) (19.2237, -25.1315) (19.2248, -25.1016) (19.2257, -25.0716) (19.2265, -25.0416) (19.2271, -25.0115) (19.2275, -24.9814) (19.2278, -24.9512) (19.2279, -24.921) (19.2279, -24.8907) (19.2277, -24.8604) (19.2273, -24.8301) (19.2268, -24.7997) (19.2261, -24.7693) (19.2253, -24.7388) (19.2243, -24.7083) (19.2232, -24.6777) (19.2219, -24.6471) (19.2205, -24.6165) (19.2189, -24.5858) (19.2172, -24.5551) (19.2153, -24.5244) (19.2132, -24.4936) (19.2111, -24.4628) (19.2087, -24.4319) (19.2063, -24.401) (19.2036, -24.3701) (19.2009, -24.3392) (19.198, -24.3082) (19.1949, -24.2772) (19.1917, -24.2462) (19.1884, -24.2151) (19.1849, -24.184) (19.182, -24.1591) (19.1798, -24.1404) (19.1783, -24.128) (19.1775, -24.1217) knots 0 0 0 0 0 0 0.01428571 0.02857143 0.04285714 0.05714286 0.07142857 0.08571429 0.1 0.11428571 0.12857143 0.14285714 0.15714286 0.17142857 0.18571429 0.2 0.21428571 0.22857143 0.24285714 0.25714286 0.27142857 0.28571429 0.3 0.31428571 0.32857143 0.34285714 0.35714286 0.37142857 0.38571429 0.4 0.41428571 0.42857143 0.44285714 0.45714286 0.47142857 0.48571429 0.5 0.51428571 0.52857143 0.54285714 0.55714286 0.57142857 0.58571429 0.6 0.61428571 0.62857143 0.64285714 0.65714286 0.67142857 0.68571429 0.7 0.71428571 0.72857143 0.74285714 0.75714286 0.77142857 0.78571429 0.8 0.81428571 0.82857143 0.84285714 0.85714286 0.87142857 0.88571429 0.9 0.91428571 0.92857143 0.94285714 0.95714286 0.97142857 0.98571429 1 1 1 1 1 1
  arc A50 (19.1775, -24.1217) -> (18.4274, -23.8298) centre (13.5, -37.5997) ccw
  spline S25 degree 5 poles (17.1374, -25.4465) (17.139, -25.4411) (17.1424, -25.4303) (17.1479, -25.4143) (17.1559, -25.3931) (17.167, -25.3671) (17.1789, -25.3413) (17.1912, -25.3157) (17.2038, -25.2901) (17.2166, -25.2646) (17.2295, -25.2392) (17.2427, -25.2138) (17.2562, -25.1886) (17.27, -25.1635) (17.2842, -25.1385) (17.2988, -25.1136) (17.3136, -25.0889) (17.3287, -25.0642) (17.344, -25.0397) (17.3595, -25.0152) (17.3751, -24.9908) (17.391, -24.9664) (17.4071, -24.9422) (17.4235, -24.9181) (17.44, -24.894) (17.4568, -24.87) (17.4738, -24.8461) (17.4909, -24.8223) (17.5083, -24.7986) (17.5258, -24.7749) (17.5435, -24.7514) (17.5614, -24.7279) (17.5795, -24.7044) (17.5977, -24.6811) (17.6162, -24.6579) (17.6348, -24.6347) (17.6535, -24.6116) (17.6725, -24.5885) (17.6916, -24.5656) (17.7108, -24.5427) (17.7302, -24.5199) (17.7498, -24.4972) (17.7695, -24.4745) (17.7894, -24.452) (17.8095, -24.4295) (17.8296, -24.4071) (17.85, -24.3847) (17.8705, -24.3624) (17.8911, -24.3402) (17.9119, -24.3181) (17.9328, -24.2961) (17.9539, -24.2741) (17.9751, -24.2522) (17.9965, -24.2304) (18.0179, -24.2086) (18.0396, -24.1869) (18.0613, -24.1653) (18.0832, -24.1438) (18.1053, -24.1224) (18.1275, -24.101) (18.1498, -24.0797) (18.1722, -24.0584) (18.1948, -24.0373) (18.2175, -24.0162) (18.2403, -23.9952) (18.2632, -23.9742) (18.2863, -23.9534) (18.3095, -23.9326) (18.3329, -23.9119) (18.3563, -23.8912) (18.3799, -23.8707) (18.3989, -23.8543) (18.4131, -23.842) (18.4227, -23.8339) (18.4274, -23.8298) knots 0 0 0 0 0 0 0.01428571 0.02857143 0.04285714 0.05714286 0.07142857 0.08571429 0.1 0.11428571 0.12857143 0.14285714 0.15714286 0.17142857 0.18571429 0.2 0.21428571 0.22857143 0.24285714 0.25714286 0.27142857 0.28571429 0.3 0.31428571 0.32857143 0.34285714 0.35714286 0.37142857 0.38571429 0.4 0.41428571 0.42857143 0.44285714 0.45714286 0.47142857 0.48571429 0.5 0.51428571 0.52857143 0.54285714 0.55714286 0.57142857 0.58571429 0.6 0.61428571 0.62857143 0.64285714 0.65714286 0.67142857 0.68571429 0.7 0.71428571 0.72857143 0.74285714 0.75714286 0.77142857 0.78571429 0.8 0.81428571 0.82857143 0.84285714 0.85714286 0.87142857 0.88571429 0.9 0.91428571 0.92857143 0.94285714 0.95714286 0.97142857 0.98571429 1 1 1 1 1 1
  line L25 (17.1374, -25.4465) -> (16.9971, -25.9131)
  arc A51 (16.8734, -25.9803) -> (16.9971, -25.9131) centre (16.9013, -25.8843) ccw
  arc A52 (16.8734, -25.9803) -> (15.8797, -25.7368) centre (13.5, -37.5997) ccw
  arc A53 (15.8011, -25.6201) -> (15.8797, -25.7368) centre (15.8993, -25.6388) ccw
  line L26 (15.8011, -25.6201) -> (15.8923, -25.1415)
  spline S26 degree 5 poles (15.8923, -25.1415) (15.8934, -25.1359) (15.8954, -25.1248) (15.8979, -25.108) (15.9006, -25.0856) (15.9028, -25.0573) (15.9042, -25.029) (15.9051, -25.0006) (15.9058, -24.9721) (15.9062, -24.9436) (15.9065, -24.9151) (15.9065, -24.8865) (15.9062, -24.8579) (15.9056, -24.8292) (15.9045, -24.8005) (15.9031, -24.7717) (15.9014, -24.7429) (15.8994, -24.7141) (15.8972, -24.6852) (15.8948, -24.6564) (15.8922, -24.6275) (15.8893, -24.5985) (15.8863, -24.5696) (15.8829, -24.5406) (15.8794, -24.5116) (15.8756, -24.4826) (15.8716, -24.4536) (15.8674, -24.4245) (15.8629, -24.3955) (15.8583, -24.3664) (15.8535, -24.3373) (15.8485, -24.3082) (15.8433, -24.2791) (15.8379, -24.25) (15.8323, -24.2208) (15.8266, -24.1917) (15.8206, -24.1625) (15.8145, -24.1333) (15.8081, -24.1042) (15.8016, -24.075) (15.795, -24.0458) (15.7881, -24.0166) (15.7811, -23.9874) (15.7739, -23.9582) (15.7665, -23.929) (15.759, -23.8997) (15.7513, -23.8705) (15.7434, -23.8413) (15.7354, -23.8121) (15.7272, -23.7829) (15.7188, -23.7536) (15.7103, -23.7244) (15.7016, -23.6952) (15.6927, -23.666) (15.6837, -23.6367) (15.6746, -23.6075) (15.6653, -23.5783) (15.6558, -23.5491) (15.6462, -23.5199) (15.6364, -23.4907) (15.6265, -23.4615) (15.6164, -23.4323) (15.6061, -23.4031) (15.5958, -23.3739) (15.5852, -23.3447) (15.5746, -23.3155) (15.5637, -23.2864) (15.5528, -23.2572) (15.5416, -23.228) (15.5304, -23.1989) (15.519, -23.1698) (15.5097, -23.1465) (15.5028, -23.129) (15.4981, -23.1173) (15.4957, -23.1115) knots 0 0 0 0 0 0 0.01428571 0.02857143 0.04285714 0.05714286 0.07142857 0.08571429 0.1 0.11428571 0.12857143 0.14285714 0.15714286 0.17142857 0.18571429 0.2 0.21428571 0.22857143 0.24285714 0.25714286 0.27142857 0.28571429 0.3 0.31428571 0.32857143 0.34285714 0.35714286 0.37142857 0.38571429 0.4 0.41428571 0.42857143 0.44285714 0.45714286 0.47142857 0.48571429 0.5 0.51428571 0.52857143 0.54285714 0.55714286 0.57142857 0.58571429 0.6 0.61428571 0.62857143 0.64285714 0.65714286 0.67142857 0.68571429 0.7 0.71428571 0.72857143 0.74285714 0.75714286 0.77142857 0.78571429 0.8 0.81428571 0.82857143 0.84285714 0.85714286 0.87142857 0.88571429 0.9 0.91428571 0.92857143 0.94285714 0.95714286 0.97142857 0.98571429 1 1 1 1 1 1
  arc A54 (15.4957, -23.1115) -> (14.6956, -23.0237) centre (13.5, -37.5997) ccw
  spline S27 degree 5 poles (13.868, -24.9192) (13.8681, -24.9135) (13.8686, -24.9022) (13.8698, -24.8853) (13.8721, -24.8628) (13.876, -24.8348) (13.8808, -24.8068) (13.8861, -24.7789) (13.8916, -24.7509) (13.8974, -24.723) (13.9033, -24.6951) (13.9095, -24.6672) (13.9159, -24.6393) (13.9228, -24.6115) (13.9301, -24.5837) (13.9377, -24.5559) (13.9456, -24.5282) (13.9538, -24.5005) (13.9622, -24.4728) (13.9708, -24.4451) (13.9797, -24.4175) (13.9887, -24.3898) (13.998, -24.3623) (14.0075, -24.3347) (14.0173, -24.3072) (14.0273, -24.2797) (14.0375, -24.2522) (14.0479, -24.2248) (14.0585, -24.1974) (14.0694, -24.17) (14.0804, -24.1426) (14.0916, -24.1153) (14.103, -24.088) (14.1145, -24.0607) (14.1263, -24.0335) (14.1383, -24.0063) (14.1504, -23.9791) (14.1627, -23.952) (14.1753, -23.9249) (14.1879, -23.8978) (14.2008, -23.8707) (14.2138, -23.8437) (14.227, -23.8167) (14.2404, -23.7898) (14.2539, -23.7629) (14.2676, -23.736) (14.2815, -23.7091) (14.2955, -23.6823) (14.3097, -23.6555) (14.324, -23.6288) (14.3385, -23.6021) (14.3532, -23.5754) (14.368, -23.5488) (14.383, -23.5221) (14.3981, -23.4956) (14.4134, -23.469) (14.4288, -23.4425) (14.4444, -23.4161) (14.4602, -23.3896) (14.476, -23.3633) (14.4921, -23.3369) (14.5083, -23.3106) (14.5246, -23.2843) (14.541, -23.2581) (14.5576, -23.2319) (14.5744, -23.2057) (14.5913, -23.1796) (14.6083, -23.1535) (14.6255, -23.1274) (14.6428, -23.1014) (14.6603, -23.0755) (14.6743, -23.0547) (14.685, -23.0392) (14.6921, -23.0288) (14.6956, -23.0237) knots 0 0 0 0 0 0 0.01428571 0.02857143 0.04285714 0.05714286 0.07142857 0.08571429 0.1 0.11428571 0.12857143 0.14285714 0.15714286 0.17142857 0.18571429 0.2 0.21428571 0.22857143 0.24285714 0.25714286 0.27142857 0.28571429 0.3 0.31428571 0.32857143 0.34285714 0.35714286 0.37142857 0.38571429 0.4 0.41428571 0.42857143 0.44285714 0.45714286 0.47142857 0.48571429 0.5 0.51428571 0.52857143 0.54285714 0.55714286 0.57142857 0.58571429 0.6 0.61428571 0.62857143 0.64285714 0.65714286 0.67142857 0.68571429 0.7 0.71428571 0.72857143 0.74285714 0.75714286 0.77142857 0.78571429 0.8 0.81428571 0.82857143 0.84285714 0.85714286 0.87142857 0.88571429 0.9 0.91428571 0.92857143 0.94285714 0.95714286 0.97142857 0.98571429 1 1 1 1 1 1
  line L27 (13.868, -24.9192) -> (13.8532, -25.4062)
  arc A55 (13.7512, -25.5031) -> (13.8532, -25.4062) centre (13.7532, -25.4031) ccw
  arc A56 (13.7512, -25.5031) -> (12.7282, -25.5252) centre (13.5, -37.5997) ccw
  arc A57 (12.6221, -25.4327) -> (12.7282, -25.5252) centre (12.7219, -25.4254) ccw
  line L28 (12.6221, -25.4327) -> (12.5864, -24.9468)
  spline S28 degree 5 poles (12.5864, -24.9468) (12.586, -24.9412) (12.585, -24.9299) (12.5831, -24.913) (12.5799, -24.8907) (12.5747, -24.8628) (12.5687, -24.8351) (12.5623, -24.8074) (12.5555, -24.7797) (12.5486, -24.7521) (12.5415, -24.7244) (12.5341, -24.6968) (12.5264, -24.6692) (12.5183, -24.6417) (12.5099, -24.6143) (12.5011, -24.5868) (12.492, -24.5595) (12.4826, -24.5321) (12.473, -24.5048) (12.4632, -24.4776) (12.4532, -24.4503) (12.443, -24.4231) (12.4325, -24.396) (12.4218, -24.3689) (12.4109, -24.3418) (12.3997, -24.3147) (12.3883, -24.2877) (12.3767, -24.2608) (12.3649, -24.2338) (12.3529, -24.2069) (12.3408, -24.1801) (12.3284, -24.1533) (12.3158, -24.1265) (12.3031, -24.0997) (12.2902, -24.073) (12.277, -24.0464) (12.2637, -24.0198) (12.2502, -23.9932) (12.2366, -23.9666) (12.2228, -23.9401) (12.2088, -23.9136) (12.1946, -23.8872) (12.1802, -23.8608) (12.1657, -23.8345) (12.151, -23.8082) (12.1362, -23.7819) (12.1212, -23.7557) (12.106, -23.7295) (12.0907, -23.7033) (12.0752, -23.6772) (12.0596, -23.6512) (12.0438, -23.6251) (12.0278, -23.5992) (12.0117, -23.5732) (11.9954, -23.5473) (11.979, -23.5215) (11.9625, -23.4957) (11.9458, -23.4699) (11.9289, -23.4442) (11.9119, -23.4185) (11.8947, -23.3928) (11.8774, -23.3672) (11.86, -23.3417) (11.8424, -23.3162) (11.8247, -23.2907) (11.8068, -23.2653) (11.7888, -23.2399) (11.7707, -23.2146) (11.7524, -23.1893) (11.734, -23.1641) (11.7154, -23.1389) (11.7005, -23.1188) (11.6892, -23.1037) (11.6817, -23.0937) (11.6779, -23.0887) knots 0 0 0 0 0 0 0.01428571 0.02857143 0.04285714 0.05714286 0.07142857 0.08571429 0.1 0.11428571 0.12857143 0.14285714 0.15714286 0.17142857 0.18571429 0.2 0.21428571 0.22857143 0.24285714 0.25714286 0.27142857 0.28571429 0.3 0.31428571 0.32857143 0.34285714 0.35714286 0.37142857 0.38571429 0.4 0.41428571 0.42857143 0.44285714 0.45714286 0.47142857 0.48571429 0.5 0.51428571 0.52857143 0.54285714 0.55714286 0.57142857 0.58571429 0.6 0.61428571 0.62857143 0.64285714 0.65714286 0.67142857 0.68571429 0.7 0.71428571 0.72857143 0.74285714 0.75714286 0.77142857 0.78571429 0.8 0.81428571 0.82857143 0.84285714 0.85714286 0.87142857 0.88571429 0.9 0.91428571 0.92857143 0.94285714 0.95714286 0.97142857 0.98571429 1 1 1 1 1 1
  arc A58 (11.6779, -23.0887) -> (10.8823, -23.2109) centre (13.5, -37.5997) ccw
  spline S29 degree 5 poles (10.5735, -25.256) (10.5722, -25.2505) (10.5697, -25.2395) (10.5664, -25.2229) (10.5629, -25.2005) (10.5594, -25.1724) (10.5568, -25.1442) (10.5546, -25.1158) (10.5528, -25.0874) (10.5511, -25.0589) (10.5496, -25.0304) (10.5483, -25.0019) (10.5474, -24.9733) (10.5468, -24.9446) (10.5466, -24.9159) (10.5468, -24.8871) (10.5473, -24.8582) (10.548, -24.8293) (10.549, -24.8004) (10.5501, -24.7715) (10.5515, -24.7425) (10.5531, -24.7135) (10.5549, -24.6844) (10.557, -24.6553) (10.5593, -24.6262) (10.5618, -24.5971) (10.5646, -24.5679) (10.5676, -24.5387) (10.5707, -24.5095) (10.5741, -24.4802) (10.5776, -24.4509) (10.5814, -24.4217) (10.5853, -24.3923) (10.5894, -24.363) (10.5938, -24.3336) (10.5983, -24.3043) (10.603, -24.2749) (10.6079, -24.2455) (10.6129, -24.2161) (10.6182, -24.1866) (10.6236, -24.1572) (10.6292, -24.1277) (10.6349, -24.0982) (10.6409, -24.0687) (10.647, -24.0392) (10.6533, -24.0097) (10.6597, -23.9802) (10.6663, -23.9507) (10.6731, -23.9211) (10.68, -23.8916) (10.6871, -23.862) (10.6944, -23.8324) (10.7018, -23.8029) (10.7094, -23.7733) (10.7171, -23.7437) (10.725, -23.7141) (10.733, -23.6845) (10.7413, -23.6549) (10.7496, -23.6253) (10.7581, -23.5957) (10.7668, -23.5661) (10.7756, -23.5365) (10.7846, -23.5069) (10.7937, -23.4773) (10.8029, -23.4477) (10.8123, -23.4181) (10.8219, -23.3885) (10.8316, -23.3589) (10.8415, -23.3293) (10.8514, -23.2997) (10.8616, -23.2701) (10.8698, -23.2464) (10.876, -23.2286) (10.8802, -23.2168) (10.8823, -23.2109) knots 0 0 0 0 0 0 0.01428571 0.02857143 0.04285714 0.05714286 0.07142857 0.08571429 0.1 0.11428571 0.12857143 0.14285714 0.15714286 0.17142857 0.18571429 0.2 0.21428571 0.22857143 0.24285714 0.25714286 0.27142857 0.28571429 0.3 0.31428571 0.32857143 0.34285714 0.35714286 0.37142857 0.38571429 0.4 0.41428571 0.42857143 0.44285714 0.45714286 0.47142857 0.48571429 0.5 0.51428571 0.52857143 0.54285714 0.55714286 0.57142857 0.58571429 0.6 0.61428571 0.62857143 0.64285714 0.65714286 0.67142857 0.68571429 0.7 0.71428571 0.72857143 0.74285714 0.75714286 0.77142857 0.78571429 0.8 0.81428571 0.82857143 0.84285714 0.85714286 0.87142857 0.88571429 0.9 0.91428571 0.92857143 0.94285714 0.95714286 0.97142857 0.98571429 1 1 1 1 1 1
  line L29 (10.5735, -25.256) -> (10.6852, -25.7303)
  arc A59 (10.6118, -25.8503) -> (10.6852, -25.7303) centre (10.5879, -25.7532) ccw
  arc A60 (10.6118, -25.8503) -> (9.6294, -26.1363) centre (13.5, -37.5997) ccw
  arc A61 (9.503, -26.0745) -> (9.6294, -26.1363) centre (9.5974, -26.0416) ccw
  line L30 (9.503, -26.0745) -> (9.3427, -25.6144)
  spline S30 degree 5 poles (9.3427, -25.6144) (9.3408, -25.6091) (9.337, -25.5984) (9.3308, -25.5826) (9.3219, -25.5619) (9.3097, -25.5363) (9.2967, -25.5111) (9.2833, -25.486) (9.2696, -25.461) (9.2558, -25.4361) (9.2418, -25.4112) (9.2275, -25.3865) (9.2129, -25.3618) (9.198, -25.3373) (9.1828, -25.313) (9.1672, -25.2888) (9.1513, -25.2647) (9.1351, -25.2407) (9.1188, -25.2168) (9.1023, -25.193) (9.0856, -25.1693) (9.0686, -25.1457) (9.0515, -25.1222) (9.0341, -25.0987) (9.0166, -25.0754) (8.9988, -25.0522) (8.9808, -25.029) (8.9626, -25.006) (8.9443, -24.983) (8.9257, -24.9602) (8.907, -24.9374) (8.8881, -24.9147) (8.8691, -24.8921) (8.8498, -24.8695) (8.8304, -24.8471) (8.8108, -24.8247) (8.7911, -24.8024) (8.7712, -24.7803) (8.7511, -24.7582) (8.7309, -24.7361) (8.7105, -24.7142) (8.69, -24.6923) (8.6693, -24.6705) (8.6485, -24.6489) (8.6275, -24.6272) (8.6063, -24.6057) (8.5851, -24.5843) (8.5636, -24.5629) (8.5421, -24.5416) (8.5203, -24.5204) (8.4985, -24.4993) (8.4765, -24.4782) (8.4544, -24.4573) (8.4321, -24.4364) (8.4097, -24.4156) (8.3871, -24.3948) (8.3645, -24.3742) (8.3416, -24.3536) (8.3187, -24.3331) (8.2956, -24.3127) (8.2724, -24.2924) (8.2491, -24.2722) (8.2256, -24.252) (8.2021, -24.2319) (8.1784, -24.2119) (8.1545, -24.192) (8.1306, -24.1721) (8.1065, -24.1523) (8.0823, -24.1327) (8.058, -24.113) (8.0335, -24.0935) (8.0139, -24.078) (7.9991, -24.0663) (7.9892, -24.0586) (7.9842, -24.0547) knots 0 0 0 0 0 0 0.01428571 0.02857143 0.04285714 0.05714286 0.07142857 0.08571429 0.1 0.11428571 0.12857143 0.14285714 0.15714286 0.17142857 0.18571429 0.2 0.21428571 0.22857143 0.24285714 0.25714286 0.27142857 0.28571429 0.3 0.31428571 0.32857143 0.34285714 0.35714286 0.37142857 0.38571429 0.4 0.41428571 0.42857143 0.44285714 0.45714286 0.47142857 0.48571429 0.5 0.51428571 0.52857143 0.54285714 0.55714286 0.57142857 0.58571429 0.6 0.61428571 0.62857143 0.64285714 0.65714286 0.67142857 0.68571429 0.7 0.71428571 0.72857143 0.74285714 0.75714286 0.77142857 0.78571429 0.8 0.81428571 0.82857143 0.84285714 0.85714286 0.87142857 0.88571429 0.9 0.91428571 0.92857143 0.94285714 0.95714286 0.97142857 0.98571429 1 1 1 1 1 1
  arc A62 (7.9842, -24.0547) -> (7.2474, -24.3787) centre (13.5, -37.5997) ccw